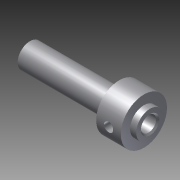
# Autodesk Inventor part: Hjulstopp
Saved by Autodesk Inventor 2012 SP1 (Build 160190100, 190)
## iProperties
Created: 2014-02-18
Part Number: Hjulstopp
Material: Default
Document SubType Name: Modeling
Designer: Pinkponk
Density: 1 g/cm^3
Author: Pinkponk
Autodesk Inventor part; units mm, degrees
ref_plane "YZ Plane" through (0, 0, 0) normal (1, 0, 0) x (0, 1, 0)
ref_plane "XZ Plane" through (0, 0, 0) normal (0, 1, 0) x (-1, 0, 0)
ref_plane "XY Plane" through (0, 0, 0) normal (0, 0, 1) x (1, 0, 0)
sketch "Sketch1" plane through (0, 0, 0) normal (0, 0, 1) x (1, 0, 0)
  line L0 (0, 0) -> (0, 4)
  line L1 (0, 4) -> (29, 4)
  line L2 (29, 4) -> (29, 7.5)
  line L3 (29, 7.5) -> (37, 7.5)
  line L4 (37, 7.5) -> (37, 4.5)
  line L5 (37, 4.5) -> (39, 4.5)
  line L6 (39, 4.5) -> (39, 2.5)
  line L7 (39, 2.5) -> (15, 2.5)
  line L8 (15, 2.5) -> (15, 0)
  line L9 (15, 0) -> (0, 0)
  line L10 (0, 0) -> (32.1678, 0)
  dimension "d0" = 8
  dimension "d1" = 39
  dimension "d2" = 15
  dimension "d3" = 8
  dimension "d4" = 2
  dimension "d5" = 9
  dimension "d6" = 5
  dimension "d7" = 15
  constraints: 22 end point, 7 parallel, 2 perpendicular, 1 collinear, 1 vertical
  measures "d0" diameter of L1 L10
  measures "d1" distance between parallel lines of L0 L6
  measures "d2" diameter of L3 L10
  measures "d3" distance between parallel lines of L4 L2
  measures "d4" distance of L4.end L5.end
  measures "d5" diameter of L5 L10
  measures "d6" diameter of L7 L10
  measures "d7" distance between parallel lines of L0 L8
revolve "Revolution1" add sketch "Sketch1" angle 360 about axis through (0, 0, 0) along (1, 0, 0)
chamfer "Chamfer1" distance 0.5 angle 45 1 edges at (39, -2.5, 0)
sketch "Sketch2" plane through (0, 0, 0) normal (0, 1, 0) x (-1, 0, 0)
  circle A0 centre (-33, 0) radius 1.5
  line L0 (0, -4) -> (-29, -4) projected
  line L1 (-29, -4) -> (-29, -7.5) projected
  line L2 (-29, -7.5) -> (-37, -7.5) projected
  line L3 (-37, -7.5) -> (-37, -4.5) projected
  line L4 (-37, -4.5) -> (-39, -4.5) projected
  line L5 (-39, -4.5) -> (-39, -3) projected
  line L6 (-39, -3) -> (-38.5, -2.5) projected
  line L7 (-38.5, -2.5) -> (-15, -2.5) projected
  line L8 (-15, -2.5) -> (-15, 2.5) projected
  line L9 (-15, 2.5) -> (-38.5, 2.5) projected
  line L10 (-38.5, 2.5) -> (-39, 3) projected
  line L11 (-39, 3) -> (-39, 4.5) projected
  line L12 (-39, 4.5) -> (-37, 4.5) projected
  line L13 (-37, 4.5) -> (-37, 7.5) projected
  line L14 (-37, 7.5) -> (-29, 7.5) projected
  line L15 (-29, 7.5) -> (-29, 4) projected
  line L16 (-29, 4) -> (0, 4) projected
  line L17 (0, 4) -> (0, -4) projected
  line L18 (-37, 7.5) -> (-37, -7.5) projected
  line L19 (-29, 7.5) -> (-29, -7.5) projected
  line L20 (-29, 4) -> (-29, -4) projected
  line L21 (0, 4) -> (0, -4) projected
  line L22 (-38.5, -2.5) -> (-38.5, 2.5) projected
  line L23 (0, -4) -> (-29, -4) projected
  point P0 (0, 0)
  point P1 (-15, 0)
  point P2 (-33, 7.5)
  dimension "d12" = 3
  constraints: 2 midpoint, 1 centre point, 1 horizontal alignment, 1 vertical alignment
  measures "d12" diameter of A0
extrude "Extrusion1" cut sketch "Sketch2" along normal through all both and the other way through all contours A0
body "Solid1"
